Autodesk Fusion 360 part; units mm, degrees
(part 3 of 3)
sketch "left.dxf" plane through (0, 0, 0) normal (-1, 0, 0) x (0, -1, 0) in component "left"
  line L0 (-57, 159) -> (-57, 156)
  line L1 (-57, 156) -> (-64.5, 156)
  line L2 (-64.5, 156) -> (-64.5, 159)
  line L3 (-64.5, 159) -> (-57, 159)
  line L4 (-18, 156) -> (-18, 159)
  line L5 (-18, 159) -> (-10.5, 159)
  line L6 (-10.5, 159) -> (-10.5, 156)
  line L7 (-10.5, 156) -> (-18, 156)
  line L8 (-64.2857, 197) -> (-72, 197)
  line L9 (-72, 197) -> (-72, 177.7778)
  line L10 (-72, 177.7778) -> (-75, 177.7778)
  line L11 (-75, 177.7778) -> (-75, 155.5556)
  line L12 (-75, 155.5556) -> (-72, 155.5556)
  line L13 (-72, 155.5556) -> (-72, 133.3333)
  line L14 (-72, 133.3333) -> (-75, 133.3333)
  line L15 (-75, 133.3333) -> (-75, 111.1111)
  line L16 (-75, 111.1111) -> (-72, 111.1111)
  line L17 (-72, 111.1111) -> (-72, 88.8889)
  line L18 (-72, 88.8889) -> (-75, 88.8889)
  line L19 (-75, 88.8889) -> (-75, 66.6667)
  line L20 (-75, 66.6667) -> (-72, 66.6667)
  line L21 (-72, 66.6667) -> (-72, 44.4444)
  line L22 (-72, 44.4444) -> (-75, 44.4444)
  line L23 (-75, 44.4444) -> (-75, 22.2222)
  line L24 (-75, 22.2222) -> (-72, 22.2222)
  line L25 (-72, 22.2222) -> (-72, 3)
  line L26 (-72, 3) -> (-64.2857, 3)
  line L27 (-64.2857, 3) -> (-64.2857, 0)
  line L28 (-64.2857, 0) -> (-53.5714, 0)
  line L29 (-53.5714, 0) -> (-53.5714, 3)
  line L30 (-53.5714, 3) -> (-42.8571, 3)
  line L31 (-42.8571, 3) -> (-42.8571, 0)
  line L32 (-42.8571, 0) -> (-32.1429, 0)
  line L33 (-32.1429, 0) -> (-32.1429, 3)
  line L34 (-32.1429, 3) -> (-21.4286, 3)
  line L35 (-21.4286, 3) -> (-21.4286, 0)
  line L36 (-21.4286, 0) -> (-10.7143, 0)
  line L37 (-10.7143, 0) -> (-10.7143, 3)
  line L38 (-10.7143, 3) -> (-3, 3)
  line L39 (-3, 3) -> (-3, 22.2222)
  line L40 (-3, 22.2222) -> (0, 22.2222)
  line L41 (0, 22.2222) -> (0, 44.4444)
  line L42 (0, 44.4444) -> (-3, 44.4444)
  line L43 (-3, 44.4444) -> (-3, 66.6667)
  line L44 (-3, 66.6667) -> (0, 66.6667)
  line L45 (0, 66.6667) -> (0, 88.8889)
  line L46 (0, 88.8889) -> (-3, 88.8889)
  line L47 (-3, 88.8889) -> (-3, 111.1111)
  line L48 (-3, 111.1111) -> (0, 111.1111)
  line L49 (0, 111.1111) -> (0, 133.3333)
  line L50 (0, 133.3333) -> (-3, 133.3333)
  line L51 (-3, 133.3333) -> (-3, 155.5556)
  line L52 (-3, 155.5556) -> (0, 155.5556)
  line L53 (0, 155.5556) -> (0, 177.7778)
  line L54 (0, 177.7778) -> (-3, 177.7778)
  line L55 (-3, 177.7778) -> (-3, 197)
  line L56 (-3, 197) -> (-10.7143, 197)
  line L57 (-10.7143, 197) -> (-10.7143, 200)
  line L58 (-10.7143, 200) -> (-21.4286, 200)
  line L59 (-21.4286, 200) -> (-21.4286, 197)
  line L60 (-21.4286, 197) -> (-32.1429, 197)
  line L61 (-32.1429, 197) -> (-32.1429, 200)
  line L62 (-32.1429, 200) -> (-42.8571, 200)
  line L63 (-42.8571, 200) -> (-42.8571, 197)
  line L64 (-42.8571, 197) -> (-53.5714, 197)
  line L65 (-53.5714, 197) -> (-53.5714, 200)
  line L66 (-53.5714, 200) -> (-64.2857, 200)
  line L67 (-64.2857, 200) -> (-64.2857, 197)
  circle A0 centre (-60, 117) radius 2.5
  line L68 (-22.5, 156) -> (-22.5, 130)
  line L69 (-22.5, 130) -> (-22.5, 127)
  line L70 (-22.5, 127) -> (-32.1429, 127)
  line L71 (-32.1429, 127) -> (-32.1429, 130)
  line L72 (-32.1429, 130) -> (-42.8571, 130)
  line L73 (-42.8571, 130) -> (-42.8571, 127)
  line L74 (-42.8571, 127) -> (-52.5, 127)
  line L75 (-52.5, 127) -> (-52.5, 130)
  line L76 (-52.5, 130) -> (-52.5, 156)
  line L77 (-52.5, 156) -> (-22.5, 156)
sketch "front.dxf" plane through (0, 0, 0) normal (0, -1, 0) x (1, 0, 0) in component "front"
  line L0 (52.5, 156) -> (52.5, 130)
  line L1 (52.5, 130) -> (50, 130)
  line L2 (50, 130) -> (50, 127)
  line L3 (50, 127) -> (41.6667, 127)
  line L4 (41.6667, 127) -> (41.6667, 130)
  line L5 (41.6667, 130) -> (33.3333, 130)
  line L6 (33.3333, 130) -> (33.3333, 127)
  line L7 (33.3333, 127) -> (25, 127)
  line L8 (25, 127) -> (25, 130)
  line L9 (25, 130) -> (22.5, 130)
  line L10 (22.5, 130) -> (22.5, 156)
  line L11 (22.5, 156) -> (52.5, 156)
  circle A0 centre (18, 117) radius 2.5
  line L12 (75, 197) -> (66.6667, 197)
  line L13 (66.6667, 197) -> (66.6667, 200)
  line L14 (66.6667, 200) -> (58.3333, 200)
  line L15 (58.3333, 200) -> (58.3333, 197)
  line L16 (58.3333, 197) -> (50, 197)
  line L17 (50, 197) -> (50, 200)
  line L18 (50, 200) -> (41.6667, 200)
  line L19 (41.6667, 200) -> (41.6667, 197)
  line L20 (41.6667, 197) -> (33.3333, 197)
  line L21 (33.3333, 197) -> (33.3333, 200)
  line L22 (33.3333, 200) -> (25, 200)
  line L23 (25, 200) -> (25, 197)
  line L24 (25, 197) -> (16.6667, 197)
  line L25 (16.6667, 197) -> (16.6667, 200)
  line L26 (16.6667, 200) -> (8.3333, 200)
  line L27 (8.3333, 200) -> (8.3333, 197)
  line L28 (8.3333, 197) -> (0, 197)
  line L29 (0, 197) -> (0, 177.7778)
  line L30 (0, 177.7778) -> (3, 177.7778)
  line L31 (3, 177.7778) -> (3, 155.5556)
  line L32 (3, 155.5556) -> (0, 155.5556)
  line L33 (0, 155.5556) -> (0, 133.3333)
  line L34 (0, 133.3333) -> (3, 133.3333)
  line L35 (3, 133.3333) -> (3, 111.1111)
  line L36 (3, 111.1111) -> (0, 111.1111)
  line L37 (0, 111.1111) -> (0, 88.8889)
  line L38 (0, 88.8889) -> (3, 88.8889)
  line L39 (3, 88.8889) -> (3, 66.6667)
  line L40 (3, 66.6667) -> (0, 66.6667)
  line L41 (0, 66.6667) -> (0, 44.4444)
  line L42 (0, 44.4444) -> (3, 44.4444)
  line L43 (3, 44.4444) -> (3, 22.2222)
  line L44 (3, 22.2222) -> (0, 22.2222)
  line L45 (0, 22.2222) -> (0, 3)
  line L46 (0, 3) -> (8.3333, 3)
  line L47 (8.3333, 3) -> (8.3333, 0)
  line L48 (8.3333, 0) -> (16.6667, 0)
  line L49 (16.6667, 0) -> (16.6667, 3)
  line L50 (16.6667, 3) -> (25, 3)
  line L51 (25, 3) -> (25, 0)
  line L52 (25, 0) -> (33.3333, 0)
  line L53 (33.3333, 0) -> (33.3333, 3)
  line L54 (33.3333, 3) -> (41.6667, 3)
  line L55 (41.6667, 3) -> (41.6667, 0)
  line L56 (41.6667, 0) -> (50, 0)
  line L57 (50, 0) -> (50, 3)
  line L58 (50, 3) -> (58.3333, 3)
  line L59 (58.3333, 3) -> (58.3333, 0)
  line L60 (58.3333, 0) -> (66.6667, 0)
  line L61 (66.6667, 0) -> (66.6667, 3)
  line L62 (66.6667, 3) -> (75, 3)
  line L63 (75, 3) -> (75, 22.2222)
  line L64 (75, 22.2222) -> (72, 22.2222)
  line L65 (72, 22.2222) -> (72, 44.4444)
  line L66 (72, 44.4444) -> (75, 44.4444)
  line L67 (75, 44.4444) -> (75, 66.6667)
  line L68 (75, 66.6667) -> (72, 66.6667)
  line L69 (72, 66.6667) -> (72, 88.8889)
  line L70 (72, 88.8889) -> (75, 88.8889)
  line L71 (75, 88.8889) -> (75, 111.1111)
  line L72 (75, 111.1111) -> (72, 111.1111)
  line L73 (72, 111.1111) -> (72, 133.3333)
  line L74 (72, 133.3333) -> (75, 133.3333)
  line L75 (75, 133.3333) -> (75, 155.5556)
  line L76 (75, 155.5556) -> (72, 155.5556)
  line L77 (72, 155.5556) -> (72, 177.7778)
  line L78 (72, 177.7778) -> (75, 177.7778)
  line L79 (75, 177.7778) -> (75, 197)
sketch "Sketch11" plane through (75, 0, 0) normal (1, 0, 0) x (0, 1, 0) in component "right"
  line L0 (64.5, 159) -> (64.5, 156)
  line L1 (64.5, 156) -> (57, 156)
  line L2 (57, 156) -> (57, 159)
  line L3 (57, 159) -> (64.5, 159)
  line L4 (10.5, 156) -> (10.5, 159)
  line L5 (10.5, 159) -> (18, 159)
  line L6 (18, 159) -> (18, 156)
  line L7 (18, 156) -> (10.5, 156)
  line L8 (52.5, 156) -> (52.5, 127)
  line L9 (52.5, 127) -> (42.8571, 127)
  line L10 (42.8571, 127) -> (42.8571, 130)
  line L11 (42.8571, 130) -> (32.1429, 130)
  line L12 (32.1429, 130) -> (32.1429, 127)
  line L13 (32.1429, 127) -> (22.5, 127)
  line L14 (22.5, 127) -> (22.5, 156)
  line L15 (22.5, 156) -> (52.5, 156)
  circle A0 centre (60, 117) radius 2.5
  line L16 (72, 197) -> (64.2857, 197)
  line L17 (64.2857, 197) -> (64.2857, 200)
  line L18 (64.2857, 200) -> (53.5714, 200)
  line L19 (53.5714, 200) -> (53.5714, 197)
  line L20 (53.5714, 197) -> (42.8571, 197)
  line L21 (42.8571, 197) -> (42.8571, 200)
  line L22 (42.8571, 200) -> (32.1429, 200)
  line L23 (32.1429, 200) -> (32.1429, 197)
  line L24 (32.1429, 197) -> (21.4286, 197)
  line L25 (21.4286, 197) -> (21.4286, 200)
  line L26 (21.4286, 200) -> (10.7143, 200)
  line L27 (10.7143, 200) -> (10.7143, 197)
  line L28 (10.7143, 197) -> (3, 197)
  line L29 (3, 197) -> (3, 177.7778)
  line L30 (3, 177.7778) -> (0, 177.7778)
  line L31 (0, 177.7778) -> (0, 155.5556)
  line L32 (0, 155.5556) -> (3, 155.5556)
  line L33 (3, 155.5556) -> (3, 133.3333)
  line L34 (3, 133.3333) -> (0, 133.3333)
  line L35 (0, 133.3333) -> (0, 111.1111)
  line L36 (0, 111.1111) -> (3, 111.1111)
  line L37 (3, 111.1111) -> (3, 88.8889)
  line L38 (3, 88.8889) -> (0, 88.8889)
  line L39 (0, 88.8889) -> (0, 66.6667)
  line L40 (0, 66.6667) -> (3, 66.6667)
  line L41 (3, 66.6667) -> (3, 44.4444)
  line L42 (3, 44.4444) -> (0, 44.4444)
  line L43 (0, 44.4444) -> (0, 22.2222)
  line L44 (0, 22.2222) -> (3, 22.2222)
  line L45 (3, 22.2222) -> (3, 3)
  line L46 (3, 3) -> (10.7143, 3)
  line L47 (10.7143, 3) -> (10.7143, 0)
  line L48 (10.7143, 0) -> (21.4286, 0)
  line L49 (21.4286, 0) -> (21.4286, 3)
  line L50 (21.4286, 3) -> (32.1429, 3)
  line L51 (32.1429, 3) -> (32.1429, 0)
  line L52 (32.1429, 0) -> (42.8571, 0)
  line L53 (42.8571, 0) -> (42.8571, 3)
  line L54 (42.8571, 3) -> (53.5714, 3)
  line L55 (53.5714, 3) -> (53.5714, 0)
  line L56 (53.5714, 0) -> (64.2857, 0)
  line L57 (64.2857, 0) -> (64.2857, 3)
  line L58 (64.2857, 3) -> (72, 3)
  line L59 (72, 3) -> (72, 22.2222)
  line L60 (72, 22.2222) -> (75, 22.2222)
  line L61 (75, 22.2222) -> (75, 44.4444)
  line L62 (75, 44.4444) -> (72, 44.4444)
  line L63 (72, 44.4444) -> (72, 66.6667)
  line L64 (72, 66.6667) -> (75, 66.6667)
  line L65 (75, 66.6667) -> (75, 88.8889)
  line L66 (75, 88.8889) -> (72, 88.8889)
  line L67 (72, 88.8889) -> (72, 111.1111)
  line L68 (72, 111.1111) -> (75, 111.1111)
  line L69 (75, 111.1111) -> (75, 133.3333)
  line L70 (75, 133.3333) -> (72, 133.3333)
  line L71 (72, 133.3333) -> (72, 155.5556)
  line L72 (72, 155.5556) -> (75, 155.5556)
  line L73 (75, 155.5556) -> (75, 177.7778)
  line L74 (75, 177.7778) -> (72, 177.7778)
  line L75 (72, 177.7778) -> (72, 197)
  line L76 (75, 44.4444) -> (75, 66.6667)
  line L77 (75, 78) -> (72, 78)
  line L78 (72, 78) -> (72, 0)
  line L79 (72, 0) -> (75, 0)
  line L80 (75, 0) -> (75, 78)
  line L81 (81.089, 0) -> (-6.089, 0)
  dimension "d322" = 3
  dimension "d323" = 78
  constraint horizontal L77
  constraint vertical L78
  constraint horizontal L79
  constraint vertical L80
  constraint coincident L65 L77.start
  constraint coincident L78.end L81
  measures "d322" distance of L77.start L77.end
  measures "d323" distance of L77.end L78.end
extrude "Extrude11" add sketch "Sketch11" against normal blind 3 contours L64 L65 L77 L78 L80 | L62 L63 L64 L76 L78 L80 | L60 L61 L62 L78 L80 | L59 L60 L78 L79 L80 L81 bodies 4 in component "right"
combine "Combine6" operation cut target body 2 tool bodies 4 keep tools in component "back"
sketch "Sketch1 (8)" plane through (0, 69, 0) normal (0, 1, 0) x (-1, 0, 0) in component "door"
  line L0 (-72, 3) -> (-66.6667, 3)
  line L1 (-66.6667, 3) -> (-66.6667, 0)
  line L2 (-66.6667, 0) -> (-58.3333, 0)
  line L3 (-58.3333, 0) -> (-58.3333, 3)
  line L4 (-58.3333, 3) -> (-50, 3)
  line L5 (-50, 3) -> (-50, 0)
  line L6 (-41.6667, 0) -> (-41.6667, 3)
  line L7 (-41.6667, 3) -> (-33.3333, 3)
  line L8 (-33.3333, 3) -> (-33.3333, 0)
  line L9 (-25, 0) -> (-25, 3)
  line L10 (-25, 3) -> (-16.6667, 3)
  line L11 (-16.6667, 3) -> (-16.6667, 0)
  line L12 (-8.3333, 0) -> (-8.3333, 3)
  line L13 (-8.3333, 3) -> (-3, 3)
  line L14 (-3, 3) -> (-3, 8)
  line L15 (-3, 8) -> (-72, 8)
  line L16 (-72, 8) -> (-72, 3)
  line L17 (-3, 3) -> (-75, 3)
  line L18 (-75, 3) -> (-75, 78)
  line L19 (-75, 78) -> (-3, 78)
  line L20 (-3, 78) -> (-3, 3)
  circle A0 centre (-21.75, 40.5) radius 7.5
  line L21 (-21.75, 48) -> (-46.75, 48)
  line L22 (-46.75, 48) -> (-46.75, 33)
  line L23 (-46.75, 33) -> (-21.75, 33)
  line L24 (-21.75, 33) -> (-21.75, 48)
  line L25 (-50, 0) -> (-41.6667, 0)
  line L26 (-33.3333, 0) -> (-25, 0)
  line L27 (-16.6667, 0) -> (-8.3333, 0)
  point P0 (-75, 88.8889)
  dimension "d303" = 75
  dimension "d304" = 15
  dimension "d305" = 25
  dimension "d307" = 37.5
  dimension "d308" = 18.75
  constraint horizontal L17
  constraint vertical L18
  constraint horizontal L19
  constraint vertical L20
  constraint coincident L13.end L14.start
  constraint coincident L18 P0
  constraint horizontal L21
  constraint vertical L22
  constraint horizontal L23
  constraint vertical L24
  constraint coincident A0.centre L24
  constraint tangent A0 L21
  constraint tangent A0 L23
  measures "d303" distance of L13.end L19.end
  measures "d304" diameter of A0
  measures "d305" distance of L21.start L21.end
  measures "d307" distance of L17 A0.centre
  measures "d308" distance of L20 A0.centre
sketch "main.dxf" plane through (0, 0, 159) normal (0, 0, 1) x (-1, 0, 0) in component "Main"
  circle A0 centre (-37.5, -51.6392) radius 1.1
  circle A1 centre (-37.5, -23.3608) radius 1.1
  line L0 (-50, -30.3) -> (-53, -30.3)
  line L1 (-53, -30.3) -> (-53, -35.1)
  line L2 (-53, -35.1) -> (-50, -35.1)
  line L3 (-50, -35.1) -> (-50, -39.9)
  line L4 (-50, -39.9) -> (-53, -39.9)
  line L5 (-53, -39.9) -> (-53, -44.7)
  line L6 (-53, -44.7) -> (-50, -44.7)
  line L7 (-50, -44.7) -> (-50, -49.5)
  line L8 (-50, -49.5) -> (-72, -49.5)
  line L9 (-72, -49.5) -> (-72, -57)
  line L10 (-72, -57) -> (-75, -57)
  line L11 (-75, -57) -> (-75, -64.5)
  line L12 (-75, -64.5) -> (-72, -64.5)
  line L13 (-72, -64.5) -> (-72, -72)
  line L14 (-72, -72) -> (-58, -72)
  line L15 (-58, -72) -> (-58, -56.875)
  line L16 (-58, -56.875) -> (-17, -56.875)
  line L17 (-17, -56.875) -> (-17, -72)
  line L18 (-17, -72) -> (-3, -72)
  line L19 (-3, -72) -> (-3, -64.5)
  line L20 (-3, -64.5) -> (0, -64.5)
  line L21 (0, -64.5) -> (0, -57)
  line L22 (0, -57) -> (-3, -57)
  line L23 (-3, -57) -> (-3, -49.5)
  line L24 (-3, -49.5) -> (-25, -49.5)
  line L25 (-25, -49.5) -> (-25, -44.7)
  line L26 (-25, -44.7) -> (-22, -44.7)
  line L27 (-22, -44.7) -> (-22, -39.9)
  line L28 (-22, -39.9) -> (-25, -39.9)
  line L29 (-25, -39.9) -> (-25, -35.1)
  line L30 (-25, -35.1) -> (-22, -35.1)
  line L31 (-22, -35.1) -> (-22, -30.3)
  line L32 (-22, -30.3) -> (-25, -30.3)
  line L33 (-25, -30.3) -> (-25, -25.5)
  line L34 (-25, -25.5) -> (-3, -25.5)
  line L35 (-3, -25.5) -> (-3, -18)
  line L36 (-3, -18) -> (0, -18)
  line L37 (0, -18) -> (0, -10.5)
  line L38 (0, -10.5) -> (-3, -10.5)
  line L39 (-3, -10.5) -> (-3, -3)
  line L40 (-3, -3) -> (-25.5, -3)
  line L41 (-25.5, -3) -> (-25.5, -19.125)
  line L42 (-25.5, -19.125) -> (-30.3, -19.125)
  line L43 (-30.3, -19.125) -> (-30.3, -16.125)
  line L44 (-30.3, -16.125) -> (-35.1, -16.125)
  line L45 (-35.1, -16.125) -> (-35.1, -19.125)
  line L46 (-35.1, -19.125) -> (-39.9, -19.125)
  line L47 (-39.9, -19.125) -> (-39.9, -16.125)
  line L48 (-39.9, -16.125) -> (-44.7, -16.125)
  line L49 (-44.7, -16.125) -> (-44.7, -19.125)
  line L50 (-44.7, -19.125) -> (-49.5, -19.125)
  line L51 (-49.5, -19.125) -> (-49.5, -3)
  line L52 (-49.5, -3) -> (-72, -3)
  line L53 (-72, -3) -> (-72, -10.5)
  line L54 (-72, -10.5) -> (-75, -10.5)
  line L55 (-75, -10.5) -> (-75, -18)
  line L56 (-75, -18) -> (-72, -18)
  line L57 (-72, -18) -> (-72, -25.5)
  line L58 (-72, -25.5) -> (-50, -25.5)
  line L59 (-50, -25.5) -> (-50, -30.3)
  line L60 (-44, -48.875) -> (-44, -26.125)
  line L61 (-44, -26.125) -> (-31, -26.125)
  line L62 (-31, -26.125) -> (-31, -48.875)
  line L63 (-31, -48.875) -> (-44, -48.875)
sketch "Sketch2 (4)" plane through (0, 0, 130) normal (0, 0, 1) x (-1, 0, 0) in component "spout"
  line L0 (-22.5, -22.125) -> (-52.5, -22.125)
  line L1 (-52.5, -22.125) -> (-52.5, 37.875)
  line L2 (-52.5, 37.875) -> (-22.5, 37.875)
  line L3 (-22.5, 37.875) -> (-22.5, -22.125)
  line L4 (-35.1, -19.125) -> (-39.9, -19.125)
  line L5 (-49.5, -19.125) -> (-49.5, -3)
  line L6 (-37.5, -72) -> (-37.5, -22.125) construction
  line L7 (-72, -72) -> (-3, -72) construction
  dimension "d276" = 3
  dimension "d277" = 3
  dimension "d278" = 60
  constraint horizontal L0
  constraint vertical L1
  constraint horizontal L2
  constraint vertical L3
  constraint vertical L6
  constraint midpoint L6.start L7
  constraint midpoint L0 L6.end
  measures "d276" distance of L0 L4
  measures "d277" distance of L1 L5
  measures "d278" distance of L0.end L1.end
extrude "Extrude1'''''''''''" add sketch "Sketch2 (4)" along normal blind 24 separate body makes body 13 in component "spout"
chamfer "Chamfer1" distance 43 angle 28 1 edges at (37.5, -37.875, 154) measured on face at (32.5, -17.875, 154) on bodies 13 in component "spout"
shell "Shell1" thickness 3 removed faces 2 at (32.5, -9.2083, 146.3788) at (32.5, 10.7917, 154) on bodies 13 in component "spout"
fillet "Fillet1'" radius 2 1 edges at (37.5, -37.875, 130) on bodies 13 in component "spout"
chamfer "Chamfer2" distance 3 angle 45 1 edges at (37.5, -34.3703, 133) measured on face at (41.5, -36.7068, 131.7577) on bodies 13 in component "spout"
ref_plane "WorkPlane1" through (37.5, -31.3703, 133) normal (0, -0.224951, 0.97437) x (-1, 0, 0) in component "spout"
extrude "Extrude2''''''" add 1 faces at (41.5, 2.2932, 133) along direction (0, 0, 1) up to surface end surface through (37.5, -31.3703, 133) normal (0, -0.224951, 0.97437) offset 0 on bodies 13 bodies 13 in component "spout"
fillet "Fillet2" radius 2 2 edges at (52.5, 22.125, 142) (22.5, 22.125, 142) on bodies 13 in component "spout"
sketch "back.dxf" plane through (0, 75, 0) normal (0, 1, 0) x (-1, 0, 0) in component "back"
  circle A0 centre (-37.5, 117) radius 2.5
  line L0 (-13, 78) -> (-13, 8)
  line L1 (-13, 8) -> (-62, 8)
  line L2 (-62, 8) -> (-62, 78)
  line L3 (-62, 78) -> (-13, 78)
  line L4 (-72, 88.8889) -> (-72, 3)
  line L5 (-72, 3) -> (-66.6667, 3)
  line L6 (-66.6667, 3) -> (-66.6667, 0)
  line L7 (-66.6667, 0) -> (-58.3333, 0)
  line L8 (-58.3333, 0) -> (-58.3333, 3)
  line L9 (-58.3333, 3) -> (-50, 3)
  line L10 (-50, 3) -> (-50, 0)
  line L11 (-50, 0) -> (-41.6667, 0)
  line L12 (-41.6667, 0) -> (-41.6667, 3)
  line L13 (-41.6667, 3) -> (-33.3333, 3)
  line L14 (-33.3333, 3) -> (-33.3333, 0)
  line L15 (-33.3333, 0) -> (-25, 0)
  line L16 (-25, 0) -> (-25, 3)
  line L17 (-25, 3) -> (-16.6667, 3)
  line L18 (-16.6667, 3) -> (-16.6667, 0)
  line L19 (-16.6667, 0) -> (-8.3333, 0)
  line L20 (-8.3333, 0) -> (-8.3333, 3)
  line L21 (-8.3333, 3) -> (0, 3)
  line L22 (0, 3) -> (0, 22.2222)
  line L23 (0, 22.2222) -> (-3, 22.2222)
  line L24 (-3, 22.2222) -> (-3, 44.4444)
  line L25 (-3, 44.4444) -> (0, 44.4444)
  line L26 (0, 44.4444) -> (0, 66.6667)
  line L27 (0, 66.6667) -> (-3, 66.6667)
  line L28 (-3, 66.6667) -> (-3, 88.8889)
  line L29 (-3, 88.8889) -> (0, 88.8889)
  line L30 (0, 88.8889) -> (0, 111.1111)
  line L31 (0, 111.1111) -> (-3, 111.1111)
  line L32 (-3, 111.1111) -> (-3, 133.3333)
  line L33 (-3, 133.3333) -> (0, 133.3333)
  line L34 (0, 133.3333) -> (0, 155.5556)
  line L35 (0, 155.5556) -> (-3, 155.5556)
  line L36 (-3, 155.5556) -> (-3, 177.7778)
  line L37 (-3, 177.7778) -> (0, 177.7778)
  line L38 (0, 177.7778) -> (0, 197)
  line L39 (0, 197) -> (-8.3333, 197)
  line L40 (-8.3333, 197) -> (-8.3333, 200)
  line L41 (-8.3333, 200) -> (-16.6667, 200)
  line L42 (-16.6667, 200) -> (-16.6667, 197)
  line L43 (-16.6667, 197) -> (-25, 197)
  line L44 (-25, 197) -> (-25, 200)
  line L45 (-25, 200) -> (-33.3333, 200)
  line L46 (-33.3333, 200) -> (-33.3333, 197)
  line L47 (-33.3333, 197) -> (-41.6667, 197)
  line L48 (-41.6667, 197) -> (-41.6667, 200)
  line L49 (-41.6667, 200) -> (-50, 200)
  line L50 (-50, 200) -> (-50, 197)
  line L51 (-50, 197) -> (-58.3333, 197)
  line L52 (-58.3333, 197) -> (-58.3333, 200)
  line L53 (-58.3333, 200) -> (-66.6667, 200)
  line L54 (-66.6667, 200) -> (-66.6667, 197)
  line L55 (-66.6667, 197) -> (-75, 197)
  line L56 (-75, 197) -> (-75, 177.7778)
  line L57 (-75, 177.7778) -> (-72, 177.7778)
  line L58 (-72, 177.7778) -> (-72, 155.5556)
  line L59 (-72, 155.5556) -> (-75, 155.5556)
  line L60 (-75, 155.5556) -> (-75, 133.3333)
  line L61 (-75, 133.3333) -> (-72, 133.3333)
  line L62 (-72, 133.3333) -> (-72, 111.1111)
  line L63 (-72, 111.1111) -> (-75, 111.1111)
  line L64 (-75, 111.1111) -> (-75, 88.8889)
  line L65 (-75, 88.8889) -> (-72, 88.8889)
extrude "Extrude3''''''" add sketch "Sketch1 (8)" along normal blind 3 separate body contours L0 L4 L7 L10 L13 L14 L15 L16 L17 L20 | L15 L16 L17 L18 L19 L20 makes body 14 in component "door"
combine "Combine14" operation cut target body 4 tool bodies 14 keep tools in component "right"
sketch "door.dxf" plane through (0, 72, 0) normal (0, 1, 0) x (-1, 0, 0) in component "door"
  line L0 (-21.75, 33) -> (-46.75, 33)
  line L1 (-46.75, 33) -> (-46.75, 48)
  line L2 (-46.75, 48) -> (-21.75, 48)
  arc A0 (-21.75, 33) -> (-21.75, 48) centre (-21.75, 40.5) ccw
  line L3 (-3, 78) -> (-75, 78)
  line L4 (-75, 78) -> (-75, 3)
  line L5 (-75, 3) -> (-3, 3)
  line L6 (-3, 3) -> (-3, 78)
sketch "side.dxf" plane through (22, 0, 0) normal (-1, 0, 0) x (0, -1, 0) in component "side left"
  line L0 (-35.1, 156) -> (-35.1, 159)
  line L1 (-35.1, 159) -> (-30.3, 159)
  line L2 (-30.3, 159) -> (-30.3, 156)
  line L3 (-30.3, 156) -> (-35.1, 156)
  line L4 (-44.7, 156) -> (-44.7, 159)
  line L5 (-44.7, 159) -> (-39.9, 159)
  line L6 (-39.9, 159) -> (-39.9, 156)
  line L7 (-39.9, 156) -> (-44.7, 156)
  line L8 (-25.5, 162) -> (-49.5, 162)
  line L9 (-49.5, 162) -> (-49.5, 151)
  line L10 (-49.5, 151) -> (-25.5, 151)
  line L11 (-25.5, 151) -> (-25.5, 162)
combine "Combine3'" operation cut target body 1 tool bodies 4 keep tools in component "base"
sketch "base.dxf" plane through (0, 0, 3) normal (0, 0, 1) x (-1, 0, 0) in component "base"
  line L0 (-72, -10.7143) -> (-72, -21.4286)
  line L1 (-72, -21.4286) -> (-75, -21.4286)
  line L2 (-75, -21.4286) -> (-75, -10.7143)
  line L3 (-75, -10.7143) -> (-72, -10.7143)
  line L4 (-72, -32.1429) -> (-72, -42.8571)
  line L5 (-72, -42.8571) -> (-75, -42.8571)
  line L6 (-75, -42.8571) -> (-75, -32.1429)
  line L7 (-75, -32.1429) -> (-72, -32.1429)
  line L8 (-72, -53.5714) -> (-72, -64.2857)
  line L9 (-72, -64.2857) -> (-75, -64.2857)
  line L10 (-75, -64.2857) -> (-75, -53.5714)
  line L11 (-75, -53.5714) -> (-72, -53.5714)
  line L12 (-72, -72) -> (-72, -75)
  line L13 (-72, -75) -> (-75, -75)
  line L14 (-75, -75) -> (-75, -72)
  line L15 (-75, -72) -> (-72, -72)
  line L16 (-58.3333, -66) -> (-58.3333, -69)
  line L17 (-58.3333, -69) -> (-66.6667, -69)
  line L18 (-66.6667, -69) -> (-66.6667, -66)
  line L19 (-66.6667, -66) -> (-58.3333, -66)
  line L20 (-41.6667, -66) -> (-41.6667, -69)
  line L21 (-41.6667, -69) -> (-50, -69)
  line L22 (-50, -69) -> (-50, -66)
  line L23 (-50, -66) -> (-41.6667, -66)
  line L24 (-25, -66) -> (-25, -69)
  line L25 (-25, -69) -> (-33.3333, -69)
  line L26 (-33.3333, -69) -> (-33.3333, -66)
  line L27 (-33.3333, -66) -> (-25, -66)
  line L28 (-8.3333, -66) -> (-8.3333, -69)
  line L29 (-8.3333, -69) -> (-16.6667, -69)
  line L30 (-16.6667, -69) -> (-16.6667, -66)
  line L31 (-16.6667, -66) -> (-8.3333, -66)
  arc A0 (-87, 15) -> (-90, 12) centre (-87, 12) ccw
  line L32 (-90, 12) -> (-90, 6.089)
  arc A1 (-90, -81.089) -> (-90, 6.089) centre (-180, -37.5) ccw
  line L33 (-90, -81.089) -> (-90, -87)
  arc A2 (-90, -87) -> (-87, -90) centre (-87, -87) ccw
  line L34 (-87, -90) -> (-81.089, -90)
  arc A3 (6.089, -90) -> (-81.089, -90) centre (-37.5, -180) ccw
  line L35 (6.089, -90) -> (12, -90)
  arc A4 (12, -90) -> (15, -87) centre (12, -87) ccw
  line L36 (15, -87) -> (15, -81.089)
  arc A5 (15, 6.089) -> (15, -81.089) centre (105, -37.5) ccw
  line L37 (15, 6.089) -> (15, 12)
  arc A6 (15, 12) -> (12, 15) centre (12, 12) ccw
  line L38 (12, 15) -> (6.089, 15)
  arc A7 (-81.089, 15) -> (6.089, 15) centre (-37.5, 105) ccw
  line L39 (-81.089, 15) -> (-87, 15)
  line L40 (-3, -10.7143) -> (0, -10.7143)
  line L41 (0, -10.7143) -> (0, -21.4286)
  line L42 (0, -21.4286) -> (-3, -21.4286)
  line L43 (-3, -21.4286) -> (-3, -10.7143)
  line L44 (-3, -32.1429) -> (0, -32.1429)
  line L45 (0, -32.1429) -> (0, -42.8571)
  line L46 (0, -42.8571) -> (-3, -42.8571)
  line L47 (-3, -42.8571) -> (-3, -32.1429)
  line L48 (-3, -53.5714) -> (0, -53.5714)
  line L49 (0, -53.5714) -> (0, -64.2857)
  line L50 (0, -64.2857) -> (-3, -64.2857)
  line L51 (-3, -64.2857) -> (-3, -53.5714)
  line L52 (-8.3333, 0) -> (-8.3333, -3)
  line L53 (-8.3333, -3) -> (-16.6667, -3)
  line L54 (-16.6667, -3) -> (-16.6667, 0)
  line L55 (-16.6667, 0) -> (-8.3333, 0)
  line L56 (-25, 0) -> (-25, -3)
  line L57 (-25, -3) -> (-33.3333, -3)
  line L58 (-33.3333, -3) -> (-33.3333, 0)
  line L59 (-33.3333, 0) -> (-25, 0)
  line L60 (-41.6667, 0) -> (-41.6667, -3)
  line L61 (-41.6667, -3) -> (-50, -3)
  line L62 (-50, -3) -> (-50, 0)
  line L63 (-50, 0) -> (-41.6667, 0)
  line L64 (-58.3333, 0) -> (-58.3333, -3)
  line L65 (-58.3333, -3) -> (-66.6667, -3)
  line L66 (-66.6667, -3) -> (-66.6667, 0)
  line L67 (-66.6667, 0) -> (-58.3333, 0)
  line L68 (-58.3333, -72) -> (-58.3333, -75)
  line L69 (-58.3333, -75) -> (-66.6667, -75)
  line L70 (-66.6667, -75) -> (-66.6667, -72)
  line L71 (-66.6667, -72) -> (-58.3333, -72)
  line L72 (-41.6667, -72) -> (-41.6667, -75)
  line L73 (-41.6667, -75) -> (-50, -75)
  line L74 (-50, -75) -> (-50, -72)
  line L75 (-50, -72) -> (-41.6667, -72)
  line L76 (-25, -72) -> (-25, -75)
  line L77 (-25, -75) -> (-33.3333, -75)
  line L78 (-33.3333, -75) -> (-33.3333, -72)
  line L79 (-33.3333, -72) -> (-25, -72)
  line L80 (-8.3333, -72) -> (-8.3333, -75)
  line L81 (-8.3333, -75) -> (-16.6667, -75)
  line L82 (-16.6667, -75) -> (-16.6667, -72)
  line L83 (-16.6667, -72) -> (-8.3333, -72)
sketch "right.dxf" plane through (75, 0, 0) normal (1, 0, 0) x (0, 1, 0) in component "right"
  line L0 (72, 78) -> (72, 0)
  line L1 (72, 0) -> (75, 0)
  line L2 (75, 0) -> (75, 88.8889)
  line L3 (75, 88.8889) -> (72, 88.8889)
  line L4 (72, 88.8889) -> (72, 111.1111)
  line L5 (72, 111.1111) -> (75, 111.1111)
  line L6 (75, 111.1111) -> (75, 133.3333)
  line L7 (75, 133.3333) -> (72, 133.3333)
  line L8 (72, 133.3333) -> (72, 155.5556)
  line L9 (72, 155.5556) -> (75, 155.5556)
  line L10 (75, 155.5556) -> (75, 177.7778)
  line L11 (75, 177.7778) -> (72, 177.7778)
  line L12 (72, 177.7778) -> (72, 197)
  line L13 (72, 197) -> (64.2857, 197)
  line L14 (64.2857, 197) -> (64.2857, 200)
  line L15 (64.2857, 200) -> (53.5714, 200)
  line L16 (53.5714, 200) -> (53.5714, 197)
  line L17 (53.5714, 197) -> (42.8571, 197)
  line L18 (42.8571, 197) -> (42.8571, 200)
  line L19 (42.8571, 200) -> (32.1429, 200)
  line L20 (32.1429, 200) -> (32.1429, 197)
  line L21 (32.1429, 197) -> (21.4286, 197)
  line L22 (21.4286, 197) -> (21.4286, 200)
  line L23 (21.4286, 200) -> (10.7143, 200)
  line L24 (10.7143, 200) -> (10.7143, 197)
  line L25 (10.7143, 197) -> (3, 197)
  line L26 (3, 197) -> (3, 177.7778)
  line L27 (3, 177.7778) -> (0, 177.7778)
  line L28 (0, 177.7778) -> (0, 155.5556)
  line L29 (0, 155.5556) -> (3, 155.5556)
  line L30 (3, 155.5556) -> (3, 133.3333)
  line L31 (3, 133.3333) -> (0, 133.3333)
  line L32 (0, 133.3333) -> (0, 111.1111)
  line L33 (0, 111.1111) -> (3, 111.1111)
  line L34 (3, 111.1111) -> (3, 88.8889)
  line L35 (3, 88.8889) -> (0, 88.8889)
  line L36 (0, 88.8889) -> (0, 66.6667)
  line L37 (0, 66.6667) -> (3, 66.6667)
  line L38 (3, 66.6667) -> (3, 44.4444)
  line L39 (3, 44.4444) -> (0, 44.4444)
  line L40 (0, 44.4444) -> (0, 22.2222)
  line L41 (0, 22.2222) -> (3, 22.2222)
  line L42 (3, 22.2222) -> (3, 3)
  line L43 (3, 3) -> (10.7143, 3)
  line L44 (10.7143, 3) -> (10.7143, 0)
  line L45 (10.7143, 0) -> (21.4286, 0)
  line L46 (21.4286, 0) -> (21.4286, 3)
  line L47 (21.4286, 3) -> (32.1429, 3)
  line L48 (32.1429, 3) -> (32.1429, 0)
  line L49 (32.1429, 0) -> (42.8571, 0)
  line L50 (42.8571, 0) -> (42.8571, 3)
  line L51 (42.8571, 3) -> (53.5714, 3)
  line L52 (53.5714, 3) -> (53.5714, 0)
  line L53 (53.5714, 0) -> (64.2857, 0)
  line L54 (64.2857, 0) -> (64.2857, 3)
  line L55 (64.2857, 3) -> (69, 3)
  line L56 (69, 3) -> (69, 78)
  line L57 (69, 78) -> (72, 78)
  line L58 (64.5, 159) -> (64.5, 156)
  line L59 (64.5, 156) -> (57, 156)
  line L60 (57, 156) -> (57, 159)
  line L61 (57, 159) -> (64.5, 159)
  line L62 (10.5, 156) -> (10.5, 159)
  line L63 (10.5, 159) -> (18, 159)
  line L64 (18, 159) -> (18, 156)
  line L65 (18, 156) -> (10.5, 156)
  line L66 (52.5, 156) -> (52.5, 127)
  line L67 (52.5, 127) -> (42.8571, 127)
  line L68 (42.8571, 127) -> (42.8571, 130)
  line L69 (42.8571, 130) -> (32.1429, 130)
  line L70 (32.1429, 130) -> (32.1429, 127)
  line L71 (32.1429, 127) -> (22.5, 127)
  line L72 (22.5, 127) -> (22.5, 156)
  line L73 (22.5, 156) -> (52.5, 156)
  circle A0 centre (60, 117) radius 2.5
sketch "Sketch5" plane through (0, 0, 200) normal (0, 0, 1) x (-1, 0, 0) in component "cover"
  line L0 (-33.3333, -72) -> (-25, -72)
  line L1 (-25, -72) -> (-25, -75)
  line L2 (-25, -75) -> (-33.3333, -75)
  line L3 (-33.3333, -75) -> (-33.3333, -72)
  line L4 (-66.6667, -72) -> (-58.3333, -72)
  line L5 (-58.3333, -72) -> (-58.3333, -75)
  line L6 (-58.3333, -75) -> (-66.6667, -75)
  line L7 (-66.6667, -75) -> (-66.6667, -72)
  line L8 (-16.6667, -72) -> (-8.3333, -72)
  line L9 (-8.3333, -72) -> (-8.3333, -75)
  line L10 (-8.3333, -75) -> (-16.6667, -75)
  line L11 (-16.6667, -75) -> (-16.6667, -72)
  line L12 (-50, -75) -> (-50, -72)
  line L13 (-50, -72) -> (-41.6667, -72)
  line L14 (-41.6667, -72) -> (-41.6667, -75)
  line L15 (-41.6667, -75) -> (-50, -75)
  line L16 (-8.3333, 0) -> (-8.3333, -3)
  line L17 (-8.3333, -3) -> (-16.6667, -3)
  line L18 (-16.6667, -3) -> (-16.6667, 0)
  line L19 (-16.6667, 0) -> (-8.3333, 0)
  line L20 (0, -42.8571) -> (-3, -42.8571)
  line L21 (-3, -42.8571) -> (-3, -32.1429)
  line L22 (-3, -32.1429) -> (0, -32.1429)
  line L23 (0, -32.1429) -> (0, -42.8571)
  line L24 (-3, -64.2857) -> (-3, -53.5714)
  line L25 (-3, -53.5714) -> (0, -53.5714)
  line L26 (0, -53.5714) -> (0, -64.2857)
  line L27 (0, -64.2857) -> (-3, -64.2857)
  line L28 (-3, -10.7143) -> (0, -10.7143)
  line L29 (0, -10.7143) -> (0, -21.4286)
  line L30 (0, -21.4286) -> (-3, -21.4286)
  line L31 (-3, -21.4286) -> (-3, -10.7143)
  line L32 (-25, 0) -> (-25, -3)
  line L33 (-25, -3) -> (-33.3333, -3)
  line L34 (-33.3333, -3) -> (-33.3333, 0)
  line L35 (-33.3333, 0) -> (-25, 0)
  line L36 (-41.6667, -3) -> (-50, -3)
  line L37 (-50, -3) -> (-50, 0)
  line L38 (-50, 0) -> (-41.6667, 0)
  line L39 (-41.6667, 0) -> (-41.6667, -3)
  line L40 (-66.6667, -3) -> (-66.6667, 0)
  line L41 (-66.6667, 0) -> (-58.3333, 0)
  line L42 (-58.3333, 0) -> (-58.3333, -3)
  line L43 (-58.3333, -3) -> (-66.6667, -3)
  line L44 (-75, -21.4286) -> (-75, -10.7143)
  line L45 (-75, -10.7143) -> (-72, -10.7143)
  line L46 (-72, -10.7143) -> (-72, -21.4286)
  line L47 (-72, -21.4286) -> (-75, -21.4286)
  line L48 (-72, -32.1429) -> (-72, -42.8571)
  line L49 (-72, -42.8571) -> (-75, -42.8571)
  line L50 (-75, -42.8571) -> (-75, -32.1429)
  line L51 (-75, -32.1429) -> (-72, -32.1429)
  line L52 (-75, -64.2857) -> (-75, -53.5714)
  line L53 (-75, -53.5714) -> (-72, -53.5714)
  line L54 (-72, -53.5714) -> (-72, -64.2857)
  line L55 (-72, -64.2857) -> (-75, -64.2857)
  line L56 (5, -80) -> (5, 5)
  line L57 (5, 5) -> (-80, 5)
  line L58 (-80, 5) -> (-80, -80)
  line L59 (-80, -80) -> (5, -80)
  line L60 (-37.5, -80) -> (-37.5, -7.7524) construction
  circle A0 centre (-37.5, -63) radius 5
  dimension "d324" = 9
  dimension "d325" = 10
  constraint midpoint L59 L60.start
  constraint perpendicular L57 L60
  constraint coincident L60 A0.centre
  measures "d324" distance of L13 A0.centre
  measures "d325" diameter of A0
extrude "Extrude3'''''''" cut sketch "Sketch5" against normal blind 3 contours A0 bodies 8 in component "cover"
sketch "cover.dxf" plane through (0, 0, 200) normal (0, 0, 1) x (-1, 0, 0) in component "cover"
  circle A0 centre (-37.5, -63) radius 5
  line L0 (-33.3333, -72) -> (-25, -72)
  line L1 (-25, -72) -> (-25, -75)
  line L2 (-25, -75) -> (-33.3333, -75)
  line L3 (-33.3333, -75) -> (-33.3333, -72)
  line L4 (-66.6667, -72) -> (-58.3333, -72)
  line L5 (-58.3333, -72) -> (-58.3333, -75)
  line L6 (-58.3333, -75) -> (-66.6667, -75)
  line L7 (-66.6667, -75) -> (-66.6667, -72)
  line L8 (-16.6667, -72) -> (-8.3333, -72)
  line L9 (-8.3333, -72) -> (-8.3333, -75)
  line L10 (-8.3333, -75) -> (-16.6667, -75)
  line L11 (-16.6667, -75) -> (-16.6667, -72)
  line L12 (-50, -75) -> (-50, -72)
  line L13 (-50, -72) -> (-41.6667, -72)
  line L14 (-41.6667, -72) -> (-41.6667, -75)
  line L15 (-41.6667, -75) -> (-50, -75)
  line L16 (-8.3333, 0) -> (-8.3333, -3)
  line L17 (-8.3333, -3) -> (-16.6667, -3)
  line L18 (-16.6667, -3) -> (-16.6667, 0)
  line L19 (-16.6667, 0) -> (-8.3333, 0)
  line L20 (0, -42.8571) -> (-3, -42.8571)
  line L21 (-3, -42.8571) -> (-3, -32.1429)
  line L22 (-3, -32.1429) -> (0, -32.1429)
  line L23 (0, -32.1429) -> (0, -42.8571)
  line L24 (-3, -64.2857) -> (-3, -53.5714)
  line L25 (-3, -53.5714) -> (0, -53.5714)
  line L26 (0, -53.5714) -> (0, -64.2857)
  line L27 (0, -64.2857) -> (-3, -64.2857)
  line L28 (-3, -10.7143) -> (0, -10.7143)
  line L29 (0, -10.7143) -> (0, -21.4286)
  line L30 (0, -21.4286) -> (-3, -21.4286)
  line L31 (-3, -21.4286) -> (-3, -10.7143)
  line L32 (-25, 0) -> (-25, -3)
  line L33 (-25, -3) -> (-33.3333, -3)
  line L34 (-33.3333, -3) -> (-33.3333, 0)
  line L35 (-33.3333, 0) -> (-25, 0)
  line L36 (-41.6667, -3) -> (-50, -3)
  line L37 (-50, -3) -> (-50, 0)
  line L38 (-50, 0) -> (-41.6667, 0)
  line L39 (-41.6667, 0) -> (-41.6667, -3)
  line L40 (-66.6667, -3) -> (-66.6667, 0)
  line L41 (-66.6667, 0) -> (-58.3333, 0)
  line L42 (-58.3333, 0) -> (-58.3333, -3)
  line L43 (-58.3333, -3) -> (-66.6667, -3)
  line L44 (-75, -21.4286) -> (-75, -10.7143)
  line L45 (-75, -10.7143) -> (-72, -10.7143)
  line L46 (-72, -10.7143) -> (-72, -21.4286)
  line L47 (-72, -21.4286) -> (-75, -21.4286)
  line L48 (-72, -32.1429) -> (-72, -42.8571)
  line L49 (-72, -42.8571) -> (-75, -42.8571)
  line L50 (-75, -42.8571) -> (-75, -32.1429)
  line L51 (-75, -32.1429) -> (-72, -32.1429)
  line L52 (-75, -64.2857) -> (-75, -53.5714)
  line L53 (-75, -53.5714) -> (-72, -53.5714)
  line L54 (-72, -53.5714) -> (-72, -64.2857)
  line L55 (-72, -64.2857) -> (-75, -64.2857)
  line L56 (5, -80) -> (5, 5)
  line L57 (5, 5) -> (-80, 5)
  line L58 (-80, 5) -> (-80, -80)
  line L59 (-80, -80) -> (5, -80)
component "tower" placed x (1, 0, 0) y (0, 1, 0) z (0, 0, 1) at (0, 0, 0)
component "Servo support" placed x (1, 0, 0) y (0, 1, 0) z (0, 0, 1) at (0, 0, 0)
component "spout" placed x (1, 0, 0) y (0, 1, 0) z (0, 0, 1) at (0, 0, 0)
component "cover" placed x (1, 0, 0) y (0, 1, 0) z (0, 0, 1) at (0, 0, 0) in component "tower"
component "slider guide" placed x (1, 0, 0) y (0, 1, 0) z (0, 0, 1) at (0, 0, 0) in component "tower"
component "mid panel" placed x (1, 0, 0) y (0, 1, 0) z (0, 0, 1) at (0, 0, 0) in component "tower"
component "left" placed x (1, 0, 0) y (0, 1, 0) z (0, 0, 1) at (0, 0, 0) in component "tower"
component "right" placed x (1, 0, 0) y (0, 1, 0) z (0, 0, 1) at (0, 0, 0) in component "tower"
component "front" placed x (1, 0, 0) y (0, 1, 0) z (0, 0, 1) at (0, 0, 0) in component "tower"
component "back" placed x (1, 0, 0) y (0, 1, 0) z (0, 0, 1) at (0, 0, 0) in component "tower"
component "base" placed x (1, 0, 0) y (0, 1, 0) z (0, 0, 1) at (0, 0, 0) in component "tower"
component "door" placed x (1, 0, 0) y (0, 1, 0) z (0, 0, 1) at (0, 0, 0) in component "tower"
component "Main" placed x (1, 0, 0) y (0, 1, 0) z (0, 0, 1) at (0, 0, 0) in component "Servo support"
component "side right" placed x (1, 0, 0) y (0, 1, 0) z (0, 0, 1) at (0, 0, 0) in component "Servo support"
component "side front" placed x (1, 0, 0) y (0, 1, 0) z (0, 0, 1) at (0, 0, 0) in component "Servo support"
component "side left" placed x (1, 0, 0) y (0, 1, 0) z (0, 0, 1) at (0, 0, 0) in component "Servo support"
equation "length = 75 mm" comment "exterior"
equation "width = 75 mm" comment "exterior"
equation "height = 200 mm" comment "exterior"
equation "thick = 3 mm" comment "material thickness"
equation "Ltab = 4" comment "No. tab"
equation "Wtab = 3" comment "No. tab"
equation "Htab = 4" comment "No. tab"
equation "WtabWidth = width / ( ( Wtab * 2 ) + 1 )" comment "tab size"
equation "LtabWidth = length / ( ( Ltab * 2 ) + 1 )" comment "tab size"
equation "HtabWidth = height / ( ( Htab * 2 ) + 1 )" comment "tab size"
equation "baseoffset = 5 mm" comment "Base outline"
equation "d14 = length"
equation "d15 = width"
equation "d16 = baseoffset"
equation "d17 = baseoffset"
equation "d18 = thick"
equation "d20 = LtabWidth"
equation "d21 = LtabWidth"
equation "d22 = -thick"
equation "d24 = Ltab"
equation "d26 = length - LtabWidth * 3"
equation "d28 = -baseoffset"
equation "d29 = height"
equation "d30 = length"
equation "d31 = -thick"
equation "d33 = HtabWidth"
equation "d34 = HtabWidth"
equation "d35 = thick"
equation "d36 = -thick"
equation "d38 = Htab"
equation "d40 = height - HtabWidth * 3"
equation "d42 = -baseoffset"
equation "d43 = thick"
equation "d45 = thick"
equation "d46 = WtabWidth"
equation "d47 = WtabWidth"
equation "d48 = -thick"
equation "d50 = Wtab"
equation "d52 = width - WtabWidth * 3"
equation "d54 = -thick"
equation "d56 = -baseoffset - thick"
equation "d57 = thick"
equation "pot = 200 mm"
equation "d60 = pot"
equation "d62 = baseoffset * 2"
equation "d63 = -thick"
equation "spoutwidth = 30 mm"
equation "spoutcutdepth = 70 mm"
equation "d69 = spoutcutdepth"
equation "d70 = spoutwidth"
equation "d73 = spoutwidth"
equation "d74 = spoutcutdepth"
equation "d77 = spoutwidth"
equation "d78 = spoutcutdepth"
equation "d81 = WtabWidth"
equation "d82 = LtabWidth"
equation "d83 = thick"
equation "d84 = LtabWidth"
equation "d85 = LtabWidth"
equation "d86 = LtabWidth"
equation "d87 = LtabWidth"
equation "d88 = thick"
equation "d89 = WtabWidth"
equation "d90 = WtabWidth"
equation "d94 = WtabWidth"
equation "d106 = -thick"
equation "d108 = -thick"
equation "d110 = -thick"
equation "d112 = -thick"
equation "d114 = thick + 5 mm"
equation "d117 = door"
equation "d122 = -thick * 2"
equation "d124 = Ltab"
equation "d126 = length - LtabWidth * 3"
equation "d128 = thick + 5 mm"
equation "d129 = thick"
equation "d156 = -thick"
equation "d159 = -thick"
equation "d162 = -thick"
equation "d194 = -thick"
equation "Sides = 69 mm"
equation "servolength = 22.75 mm"
equation "servowidth = 13 mm"
equation "thick_acrylic = 3 mm"
equation "servotab = 5 mm"
equation "spouthole = 15 mm"
equation "offset_2 = 9 mm"
equation "slotlength = 24 mm"
equation "d199 = baseoffset"
equation "d200 = -thick"
equation "d206 = length - thick * 2"
equation "d231 = -thick_acrylic"
equation "d233 = servowidth"
equation "d234 = servolength"
equation "d236 = offset_2 + 5 mm"
equation "d237 = servotab + thick_acrylic"
equation "d238 = offset_2"
equation "d239 = slotlength"
equation "d243 = thick_acrylic"
equation "d244 = slotlength / 5"
equation "d245 = slotlength / 5"
equation "d246 = slotlength / 5"
equation "d247 = slotlength / 5"
equation "d248 = slotlength / 5"
equation "d249 = thick_acrylic"
equation "d250 = slotlength / 5"
equation "d251 = slotlength / 5"
equation "d252 = slotlength / 5"
equation "d253 = slotlength / 5"
equation "d254 = slotlength / 5"
equation "d257 = 5 mm + thick_acrylic"
equation "d258 = thick_acrylic"
equation "d261 = -thick_acrylic"
equation "d264 = thick_acrylic"
equation "d266 = ( 22.5 / 3 ) * 1 mm"
equation "d267 = thick"
equation "d270 = -thick_acrylic"
equation "spoutlength = 60 mm"
equation "d276 = thick"
equation "d277 = thick"
equation "d278 = spoutlength"
equation "spoutdepth = 24 mm"
equation "d280 = spoutdepth"
equation "d284 = thick"
equation "door = 70 mm"
equation "d297 = door + 5 mm"
equation "d301 = -thick"
equation "d303 = door + 5 mm"
equation "d307 = ( door + 5 mm ) / 2"
equation "d308 = length / 4"
equation "d315 = thick"
equation "d321 = thick_acrylic"
equation "d322 = thick"
equation "d323 = door + 5 mm + thick"
equation "d324 = offset_2"
equation "d326 = -thick"
